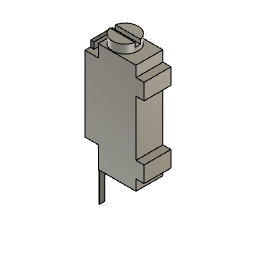
mPFC_HPC_plusminiamps (Autodesk Fusion 360 archive; units mm, degrees)
design "Nanodrive"
Autodesk Fusion 360 part; units mm, degrees
sketch "Sketch1" plane through (0, 0, 0) normal (0, 0, 1) x (1, 0, 0)
  line L0 (1.75, -1.25) -> (-1.75, -1.25)
  line L1 (-1.75, -1.25) -> (-1.75, 1.25)
  line L2 (-1.75, 1.25) -> (1.75, 1.25)
  line L3 (1.75, 1.25) -> (1.75, -1.25)
  line L4 (1.75, -1.25) -> (-1.75, 1.25) construction
  line L5 (-1.75, -1.25) -> (1.75, 1.25) construction
  dimension "d1" = 3.5
  dimension "d2" = 2.5
  constraint horizontal L0
  constraint perpendicular L0 L1
  constraint parallel L0 L2
  constraint parallel L1 L3
  constraint coincident L4 origin
  constraint coincident L5 origin
  measures "d1" distance of L1.end L2.end
  measures "d2" distance of L0.end L1.end
extrude "Extrude1" add sketch "Sketch1" along normal blind 10.16 makes body 1
sketch "Sketch2" plane through (0, 0, 10.16) normal (0, 0, 1) x (-1, 0, 0)
  line L0 (-1.75, -1.25) -> (1.75, -1.25)
  line L1 (1.75, -1.25) -> (1.75, 1.25)
  line L2 (1.75, 1.25) -> (-1.75, 1.25)
  line L3 (-1.75, 1.25) -> (-1.75, -1.25)
  circle A0 centre (0, 0) radius 1
  dimension "d5" = 2
  constraint coincident A0.centre origin
  measures "d5" diameter of A0
extrude "Extrude2" add sketch "Sketch2" along normal blind 0.8 contours A0 bodies 1
sketch "Sketch3" plane through (-1.75, 0, 0) normal (-1, 0, 0) x (0, -1, 0)
  line L0 (-1.25, 0) -> (1.25, 0)
  line L1 (1.25, 0) -> (1.25, 10.16)
  line L2 (1.25, 10.16) -> (-1.25, 10.16)
  line L3 (-1.25, 10.16) -> (-1.25, 0)
  line L4 (1.25, 2) -> (-1.25, 2)
  line L5 (-1.25, 2) -> (-1.25, 9)
  line L6 (-1.25, 9) -> (1.25, 9)
  line L7 (1.25, 9) -> (1.25, 2)
  line L8 (1.25, 2) -> (-1.25, 9) construction
  line L9 (-1.25, 2) -> (1.25, 9) construction
  point P0 (0, 5.5)
  dimension "d8" = 7
  constraint horizontal L4
  constraint perpendicular L4 L5
  constraint parallel L4 L6
  constraint parallel L5 L7
  constraint coincident L8 P0
  constraint coincident L9 P0
  measures "d8" distance of L4.end L5.end
extrude "Extrude3" add sketch "Sketch3" along normal blind 0.9 contours L1 L3 L4 L5 L6 L7 bodies 1
sketch "Sketch4" plane through (-2.65, 0, 0) normal (-1, 0, 0) x (0, -1, 0)
  line L0 (1.25, 9) -> (-1.25, 9)
  line L1 (-1.25, 9) -> (-1.25, 2)
  line L2 (-1.25, 2) -> (1.25, 2)
  line L3 (1.25, 2) -> (1.25, 9)
  line L4 (1.25, 9) -> (0.75, 9)
  line L5 (0.75, 9) -> (0.75, 2)
  line L6 (0.75, 2) -> (1.25, 2)
  line L7 (1.25, 2) -> (1.25, 9)
  dimension "d11" = 0.5
  constraint horizontal L4
  constraint vertical L5
  constraint horizontal L6
  constraint vertical L7
  constraint coincident L0.start L3.end
  measures "d11" distance of L0.start L4.end
extrude "Extrude4" add sketch "Sketch4" along normal blind 0.35 contours L0 L2 L3 L4 L5 L6 L7 bodies 1
sketch "Sketch5" plane through (1.75, 0.3805, -0.9015) normal (1, 0, 0) x (0, 1, 0)
  line L0 (-1.6305, 0.9015) -> (0.8695, 0.9015)
  line L1 (0.8695, 0.9015) -> (0.8695, 11.0615)
  line L2 (0.8695, 11.0615) -> (-1.6305, 11.0615)
  line L3 (-1.6305, 11.0615) -> (-1.6305, 0.9015)
  line L4 (-1.6305, 10.0615) -> (0.8695, 10.0615)
  line L5 (0.8695, 10.0615) -> (0.8695, 8.5615)
  line L6 (0.8695, 8.5615) -> (-1.6305, 8.5615)
  line L7 (-1.6305, 8.4708) -> (-1.6305, 9.9708)
  line L8 (-1.6305, 1.9015) -> (0.8695, 1.9015)
  line L9 (0.8695, 1.9015) -> (0.8695, 3.4015)
  line L10 (0.8695, 3.4015) -> (-1.6305, 3.4015)
  line L11 (-1.6305, 3.4015) -> (-1.6305, 1.9015)
  dimension "d14" = 1.5
  dimension "d59" = 1
  dimension "d60" = 1.5
  dimension "d61" = 1
  constraint horizontal L4
  constraint vertical L5
  constraint horizontal L6
  constraint vertical L7
  constraint coincident L1 L5.end
  constraint horizontal L8
  constraint vertical L9
  constraint horizontal L10
  constraint vertical L11
  constraint coincident L3 L8.start
  constraint collinear L3 L7
  constraint collinear L1 L9
  measures "d14" distance of L8.start L10.end
  measures "d59" distance of L0 L8
  measures "d60" distance of L4 L6
  measures "d61" distance of L2 L4
extrude "Extrude5" add sketch "Sketch5" along normal blind 0.75 contours L1 L3 L4 L5 L6 L7 bodies 1
sketch "Sketch6" plane through (1.75, 0, 0) normal (1, 0, 0) x (0, 1, 0)
  line L0 (1.25, 7.66) -> (-1.25, 7.66)
  line L1 (-1.25, 7.66) -> (-1.25, 0)
  line L2 (-1.25, 0) -> (1.25, 0)
  line L3 (1.25, 0) -> (1.25, 7.66)
  line L4 (-1.25, 0.9955) -> (1.25, 0.9955)
  line L5 (1.25, 0.9955) -> (1.25, 2.4955)
  line L6 (1.25, 2.4955) -> (-1.25, 2.4955)
  line L7 (-1.25, 2.4955) -> (-1.25, 0.9955)
  dimension "d17" = 1.5
  constraint horizontal L4
  constraint vertical L5
  constraint horizontal L6
  constraint vertical L7
  constraint coincident L1 L4.start
  measures "d17" distance of L4.start L6.end
extrude "Extrude6" add sketch "Sketch6" along normal blind 0.75 contours L1 L3 L4 L5 L6 L7 bodies 1
delete_face "DeleteFace1" 1 faces at (-0.995, 0.0996, 10.6933) on bodies 1
sketch "Sketch7" plane through (0, 0, 10.16) normal (0, 0, 1) x (-1, 0, 0)
  line L0 (-1.75, -1.25) -> (1.75, -1.25)
  line L1 (1.75, -1.25) -> (1.75, 1.25)
  line L2 (1.75, 1.25) -> (-1.75, 1.25)
  line L3 (-1.75, 1.25) -> (-1.75, -1.25)
  circle A0 centre (0.5, 0) radius 1.2
  dimension "d20" = 2.4
  measures "d20" diameter of A0
extrude "Extrude7" add sketch "Sketch7" along normal blind 0.8 contours A0 bodies 1
sketch "Sketch1 (2)" plane through (-2.65, 0, 0) normal (-1, 0, 0) x (0, -1, 0) in component "Probe"
  line L0 (0.75, 2) -> (0.75, 9.6)
  line L1 (0.75, 9.6) -> (-1.25, 9.6)
  line L2 (-1.25, 9.6) -> (-1.25, 2)
  line L3 (-1.25, 2) -> (-0.5, 2)
  line L4 (-0.5, 2) -> (-0.5, -4)
  line L5 (-0.5, -4) -> (0, -4)
  line L6 (0, -4) -> (0, 2)
  line L7 (0, 2) -> (0.75, 2)
  line L8 (-1.25, 9.6) -> (0.75, 9.6)
  line L9 (0.75, 9.6) -> (0.75, 2)
  line L10 (0.75, 2) -> (-1.25, 2)
  line L11 (-1.25, 2) -> (-1.25, 9.6)
  line L12 (0.75, 2) -> (0.75, 9)
  line L13 (0.75, 9) -> (-1.25, 9)
  line L14 (-1.25, 9) -> (-1.25, 2)
  line L15 (-1.25, 2) -> (0.75, 2)
  constraint horizontal L8
  constraint vertical L9
  constraint horizontal L10
  constraint vertical L11
  constraint coincident L0.start L7.end
  constraint coincident L1.end L2.start
extrude "Extrude1'" add sketch "Sketch1 (2)" along normal blind 0.3 separate body contours L0 L2 L3 L7 L9 L10 L11 L12 L13 L14 L15 | L0 L1 L2 L8 L9 L11 L13 makes body 2 in component "Probe"
sketch "Sketch2 (2)" plane through (0, 0, 2) normal (0, 0, -1) x (1, 0, 0) in component "Probe"
  line L0 (-2.65, -1.25) -> (-2.65, 0.75)
  line L1 (-2.65, 0.75) -> (-2.95, 0.75)
  line L2 (-2.95, 0.75) -> (-2.95, -1.25)
  line L3 (-2.95, -1.25) -> (-2.65, -1.25)
  line L4 (-2.9, -0.5) -> (-2.95, -0.5)
  line L5 (-2.95, -0.5) -> (-2.95, 0)
  line L6 (-2.95, 0) -> (-2.9, 0)
  line L7 (-2.9, 0) -> (-2.9, -0.5)
  line L8 (-2.9, -0.5) -> (-2.95, 0) construction
  line L9 (-2.95, -0.5) -> (-2.9, 0) construction
  point P0 (-2.925, -0.25)
  dimension "d53" = 0.05
  dimension "d54" = 0.5
  constraint horizontal L4
  constraint perpendicular L4 L5
  constraint parallel L4 L6
  constraint parallel L5 L7
  constraint coincident L8 P0
  constraint coincident L9 P0
  constraint collinear L2 L5
  measures "d53" distance of L5.end L6.end
  measures "d54" distance of L4.end L5.end
extrude "Extrude2'" add sketch "Sketch2 (2)" along normal blind 6 contours L2 L4 L5 L6 L7 bodies 2 in component "Probe"
sketch "Sketch8" plane through (0, 0, 10.96) normal (0, 0, 1) x (-1, 0, 0)
  circle A0 centre (0.5, 0) radius 1.2
  line L0 (1.6737, -0.25) -> (-0.6737, -0.25)
  line L1 (1.6737, 0.25) -> (-0.6737, 0.25)
  dimension "d162" = 0.5
  dimension "d163" = 0.25
  constraint coincident A0 L0.start
  constraint coincident A0 L0.end
  constraint horizontal L0
  constraint coincident A0 L1.start
  constraint coincident A0 L1.end
  constraint parallel L0 L1
  measures "d162" distance of L0 L1
  measures "d163" distance of A0.centre L0
extrude "Extrude8" cut sketch "Sketch8" against normal blind 0.4 contours A0 L0 L1 bodies 1
component "Probe" placed x (1, 0, 0) y (0, 1, 0) z (0, 0, 1) at (0, 0, 0)
named bodies: "Drive body"
